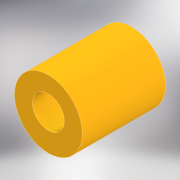
# Autodesk Inventor part: Buje
Saved by Autodesk Inventor 2021 (Build 250183000, 183)
## iProperties
Created: 2024-03-10
Part Number: Buje
Material: PLA
Document SubType Name: Modeling
Designer: Martin
Mass: 2.0935 g
Surface Area: 11.6864 cm^2
Volume: 1.64843 cm^3
Density: 1.27 g/cm^3
Appearance: PLA
Author: Martin
Autodesk Inventor part; units mm, degrees
ref_plane "YZ Plane" through (0, 0, 0) normal (1, 0, 0) x (0, 1, 0)
ref_plane "XZ Plane" through (0, 0, 0) normal (0, 1, 0) x (-1, 0, 0)
ref_plane "XY Plane" through (0, 0, 0) normal (0, 0, 1) x (1, 0, 0)
sketch "Sketch1" plane through (0, 0, 0) normal (0, 0, 1) x (1, 0, 0)
  circle A0 centre (0, 0) radius 3.075
  circle A1 centre (0, -0.3223) radius 6.5
  dimension "d0" = 6.15
  dimension "d1" = 13
  constraints: 2 centre point, 1 coincident
  measures "d0" diameter of A0
  measures "d1" diameter of A1
extrude "Extrusion1" add sketch "Sketch1" along normal blind 16
body "Solid1"
